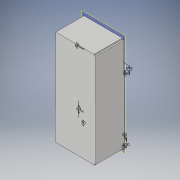
# Autodesk Inventor part: Garage
Saved by Autodesk Inventor 2017 (Build 210142000, 142)
## iProperties
Part Number: Garage
Material: Generisch
Document SubType Name: Modeling
Designer: OleSi
Density: 1 g/cm^3
Appearance: Vorgabe
Author: OleSi
Autodesk Inventor part; units mm, degrees
ref_plane "YZ Plane" through (0, 0, 0) normal (1, 0, 0) x (0, 1, 0)
ref_plane "XZ Plane" through (0, 0, 0) normal (0, 1, 0) x (-1, 0, 0)
ref_plane "XY Plane" through (0, 0, 0) normal (0, 0, 1) x (1, 0, 0)
sketch "Skizze1" plane through (0, 0, 0) normal (0, 1, 0) x (-1, 0, 0)
  line L0 (0, 0) -> (35, -6509.9059)
  line L1 (0, 0) -> (-2700, 0)
  line L2 (-2700, 0) -> (-2735, -6549.9065)
  line L3 (-2735, -6549.9065) -> (35, -6509.9059)
  line L4 (-1350, 0) -> (-1350, -6529.9062) construction
  dimension "d0" = 6510
  dimension "d1" = 2700
  dimension "d2" = 6550
  dimension "d3" = 2770
  dimension "d4" = 1350
  constraints: 10 end point, 2 midpoint, 1 horizontal, 1 vertical
  measures "d0" distance of L0.start L0.end
  measures "d1" distance of L0.start L1.end
  measures "d2" distance of L1.end L2.end
  measures "d3" horizontal distance of L2.end L0.end
  measures "d4" distance from line of L0.start L4
extrude "Extrusion1" add sketch "Skizze1" along normal blind 100
sketch "Skizze2" plane through (0, 0, 0) normal (0, 0, 1) x (1, 0, 0)
  line L0 (0, 0) -> (0, 100) projected
  line L1 (0, 0) -> (2700, 0)
  line L2 (2700, 0) -> (2700, 2000)
  line L3 (2700, 2000) -> (0, 2000)
  line L4 (0, 2000) -> (0, 0)
  dimension "d7" = 2000
  constraints: 8 end point, 2 parallel, 1 coincident, 1 horizontal, 1 perpendicular
  measures "d7" distance of L3.end L0.start
extrude "Extrusion2" add sketch "Skizze2" along normal blind 100
sketch "Skizze3" plane through (2700, 0, 0) normal (0.9999857, 0, 0.0053435) x (0.0053435, 0, -0.9999857)
  line L0 (-14.4275, 0) -> (6550, 0)
  line L1 (6550, 0) -> (6550, 2000)
  line L2 (6550, 2000) -> (-14.4275, 2000)
  line L3 (-14.4275, 2000) -> (-14.4275, 0)
  dimension "d10" = 2000
  constraints: 8 end point, 2 parallel, 1 coincident, 1 horizontal, 1 perpendicular
  measures "d10" distance of L2.end L0.start
extrude "Extrusion3" add sketch "Skizze3" along normal blind 100
sketch "Skizze4" plane through (-35, 0, -6509.9059) normal (-0.0144391, 0, -0.9998958) x (-0.9998958, 0, 0.0144391)
  line L0 (-2770.2888, 0) -> (0, 0)
  line L1 (0, 0) -> (0, 2000)
  line L2 (0, 2000) -> (-2770.2888, 2000)
  line L3 (-2770.2888, 2000) -> (-2770.2888, 0)
  line L4 (0, 0) -> (-2770.2888, 0) projected
  point P0 (59.0011, 0)
  dimension "d13" = 2000
  constraints: 8 end point, 2 parallel, 1 coincident, 1 horizontal, 1 perpendicular
  measures "d13" distance of L0.end L1.end
extrude "Extrusion4" add sketch "Skizze4" along normal blind 100
ref_plane "Arbeitsebene1" through (0, 2012, 0) normal (0, 1, 0) x (1, 0, 0)
sketch "Skizze5" plane through (0, 2012, 0) normal (0, 1, 0) x (1, 0, 0)
  line L0 (0, 0) -> (2700, 0) projected
  line L1 (0, 0) -> (2700.3741, 0)
  line L2 (2700.3741, 0) -> (2700.3741, 70)
  line L3 (2700.3741, 70) -> (-0.3763, 70)
  line L4 (-0.3763, 70) -> (0, 0)
  line L5 (2735, 6549.9065) -> (2700, 0) projected
  line L6 (-35, 6509.9059) -> (0, 0) projected
  dimension "d17" = 70
  constraints: 8 end point, 2 point on line, 1 horizontal, 1 parallel, 1 perpendicular
  measures "d17" distance of L2.end L1.end
extrude "Extrusion5" add sketch "Skizze5" along normal blind 100 contours L4 L3 L5 L0
sketch "Skizze6" plane through (0, 2012, 0) normal (0, 1, 0) x (1, 0, 0)
  line L0 (2703.7672, 705) -> (-3.7904, 705)
  line L1 (-3.7904, 705) -> (-4.113, 765)
  line L2 (-4.113, 765) -> (2704.0878, 764.9991)
  line L3 (2704.0878, 764.9991) -> (2703.7672, 705)
  line L4 (-35, 6509.9059) -> (0, 0) projected
  line L5 (2700.3741, 70) -> (-0.3763, 70) projected
  line L6 (2735, 6549.9065) -> (2700, 0) projected
  dimension "d20" = 635
  dimension "d21" = 60
  dimension "d22" = 60
  constraints: 8 end point, 4 point on line, 1 horizontal
  measures "d20" distance from line of L5 L0.start
  measures "d21" distance of L2.end L0.start
  measures "d22" vertical distance of L0.end L1.end
extrude "Extrusion6" add sketch "Skizze6" along normal blind 100 contours L0 L1 L2 L3
sketch "Skizze7" plane through (0, 2012, 0) normal (0, 1, 0) x (1, 0, 0)
  line L0 (2707.3741, 1379.9983) -> (-7.4195, 1379.9983)
  line L1 (-7.4195, 1379.9983) -> (-7.0969, 1319.9992)
  line L2 (-7.0969, 1319.9992) -> (2707.0535, 1319.9991)
  line L3 (2707.0535, 1319.9991) -> (2707.3741, 1379.9983)
  line L4 (2735, 6549.9065) -> (2700, 0) projected
  line L5 (-35, 6509.9059) -> (0, 0) projected
  line L6 (2704.0878, 764.9991) -> (-4.113, 765) projected
  dimension "d25" = 60
  dimension "d26" = 60
  dimension "d27" = 555
  constraints: 8 end point, 4 point on line, 1 horizontal
  measures "d25" distance of L2.end L0.start
  measures "d26" distance of L0.end L1.end
  measures "d27" distance from line of L6 L2.end
extrude "Extrusion7" add sketch "Skizze7" along normal blind 100 contours L3 L2 L1 L0
sketch "Skizze8" plane through (0, 2012, 0) normal (0, 1, 0) x (1, 0, 0)
  line L0 (2700, 0) -> (2735, 6549.9065) construction
  line L1 (2710.3398, 1934.9983) -> (-10.4034, 1934.9983)
  line L2 (-10.4034, 1934.9983) -> (-10.726, 1994.9983)
  line L3 (-10.726, 1994.9983) -> (2710.6604, 1994.9983)
  line L4 (2710.6604, 1994.9983) -> (2710.3398, 1934.9983)
  line L5 (-35, 6509.9059) -> (0, 0) construction
  line L6 (2707.3741, 1379.9983) -> (-7.4195, 1379.9983) projected
  line L7 (2735, 6549.9065) -> (2733.5561, 6649.8961) projected
  line L8 (2735, 6549.9065) -> (-35, 6509.9059)
  line L9 (-35, 6509.9059) -> (-34.6237, 6439.9059)
  line L10 (-34.6237, 6439.9059) -> (2734.6259, 6479.8938)
  line L11 (2734.6259, 6479.8938) -> (2735, 6549.9065)
  line L12 (2731.1525, 5829.8938) -> (-31.344, 5829.8938)
  line L13 (0, 0) -> (-35, 6509.9059) projected
  line L14 (2730.8319, 5769.8938) -> (-31.0214, 5769.8938)
  dimension "d30" = 60
  dimension "d31" = 60
  dimension "d32" = 555
  dimension "d33" = 70
  dimension "d34" = 70
  dimension "d35" = 60
  dimension "d36" = 60
  dimension "d37" = 650
  constraints: 20 end point, 10 point on line, 2 horizontal
  measures "d30" vertical distance of L1.end L2.end
  measures "d31" vertical distance of L3.end L1.start
  measures "d32" distance from line of L6 L1.start
  measures "d33" distance from line of L8 L10.end
  measures "d34" vertical distance of L5.start L9.end
  measures "d35" distance from line of L14 L12.start
  measures "d36" vertical distance of L14.end L12.end
  measures "d37" vertical distance of L10.end L12.start
equation "\"d4\" = 0.5 * d1"
